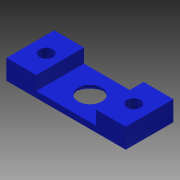
# Autodesk Inventor part: 13_1087_037
Saved by Autodesk Inventor 2014 SP1 (Build 180222100, 222)
## iProperties
Created: 2013-09-20
Part Number: 13_1087_037
Material: Allgemein
Document SubType Name: Modeling
Designer: vogel
Density: 1 g/cm^3
Appearance: Blau - Wandfarbe - glänzend
Author: vogel
Autodesk Inventor part; units mm, degrees
ref_plane "YZ Plane" through (0, 0, 0) normal (1, 0, 0) x (0, 1, 0)
ref_plane "XZ Plane" through (0, 0, 0) normal (0, 1, 0) x (-1, 0, 0)
ref_plane "XY Plane" through (0, 0, 0) normal (0, 0, 1) x (1, 0, 0)
sketch "Skizze1" plane through (0, 0, 0) normal (0, 0, 1) x (1, 0, 0)
  line L0 (-21, 0) -> (21, 0) projected
  line L1 (0, -8.4) -> (0, 8.4) projected
  line L2 (-15, 6) -> (15, 6)
  line L3 (15, 6) -> (15, -6)
  line L4 (15, -6) -> (-15, -6)
  line L5 (-15, -6) -> (-15, 6)
  point P0 (0, 0)
  dimension "d0" = 12
  dimension "d1" = 30
  constraints: 8 end point, 2 parallel, 1 horizontal, 1 perpendicular, 2 other
  measures "d0" distance of L4.end L2.start
  measures "d1" distance between parallel lines of L3 L5
extrude "Extrusion1" add sketch "Skizze1" along normal blind 5
sketch "Skizze2" plane through (0, 0, 5) normal (0, 0, 1) x (1, 0, 0)
  line L0 (15, 6) -> (-15, 6) projected
  line L1 (-15, -6) -> (15, -6) projected
  line L2 (-21, 0) -> (21, 0) projected
  line L3 (0, -8.4) -> (0, 8.4) projected
  line L4 (-7.5, 6) -> (7.5, 6)
  line L5 (7.5, 6) -> (7.5, -6)
  line L6 (7.5, -6) -> (-7.5, -6)
  line L7 (-7.5, -6) -> (-7.5, 6)
  point P0 (0, 0)
  dimension "d4" = 15
  constraints: 8 end point, 2 parallel, 2 point on line, 1 horizontal, 1 perpendicular, 1 other
  measures "d4" distance between parallel lines of L5 L7
extrude "Extrusion2" cut sketch "Skizze2" against normal blind 3.5
sketch "Skizze3" plane through (0, 0, 0) normal (0, 0, -1) x (-1, 0, 0)
  line L0 (21, 0) -> (-21, 0) projected
  line L1 (0, -8.4) -> (0, 8.4) projected
  point P0 (0, 0)
  point P1 (-11, 0)
  point P2 (11, 0)
  dimension "d7" = 22
  constraints: 2 point on line, 1 symmetric about line
  measures "d7" distance of point (11, 0) point (-11, 0)
hole "Bohrung1" at (11, 0, 0) at (-11, 0, 0) direction (0, 0, 1) diameter 3.4 end through all countersink diameter 6.9 countersink angle 90
sketch "Skizze4" plane through (0, 0, 1.5) normal (0, 0, 1) x (1, 0, 0)
  point P0 (0, 0)
  point P1 (0, 0)
  constraints: 1 coincident
hole "Bohrung2" at (0, 0, 1.5) direction (0, 0, -1) diameter 6 end through all
chamfer "Fase1" distance 1 angle 45 1 edges at (0, 3, 0)
